Autodesk Fusion 360 part; units mm, degrees
(part 7 of 25)
  arc A2551 (12.8651, 8.7313) -> (12.8651, 8.6677) centre (12.8651, 8.6995) ccw
  line L798 (13.8532, 8.0645) -> (13.8532, 9.2075)
  arc A2552 (15.5982, 8.6789) -> (15.5498, 8.7201) centre (15.574, 8.6995) ccw
  arc A2553 (13.3731, 8.0328) -> (13.3731, 8.0963) centre (13.3731, 8.0646) ccw
  arc A2554 (76.9971, 14.0193) -> (77.0539, 14.0477) centre (77.0255, 14.0335) ccw
  arc A2555 (13.8532, 9.2393) -> (13.8532, 9.1757) centre (13.8532, 9.2075) ccw
  arc A2556 (14.5199, 8.382) -> (14.4564, 8.382) centre (14.4881, 8.382) ccw
  line L799 (76.3905, 14.0335) -> (76.3905, 15.1765)
  arc A2557 (15.0041, 8.9633) -> (15.0645, 8.9437) centre (15.0343, 8.9535) ccw
  line L800 (15.0343, 8.0645) -> (15.6693, 8.0645)
  arc A2558 (76.708, 14.5415) -> (76.708, 15.1765) centre (76.708, 14.859) ccw
  arc A2559 (13.2461, 8.6677) -> (13.2461, 8.7313) centre (13.2461, 8.6995) ccw
  arc A2560 (10.8248, 9.6965) -> (10.5391, 9.9822) centre (10.5391, 9.6965) ccw
  arc A2561 (10.8566, 9.6965) -> (10.7931, 9.6964) centre (10.8249, 9.6965) ccw
  arc A2562 (76.4223, 15.1765) -> (76.3588, 15.1765) centre (76.3906, 15.1765) ccw
  arc A2563 (10.1596, 9.738) -> (10.22, 9.7184) centre (10.1898, 9.7282) ccw
  arc A2564 (10.7538, 9.4536) -> (10.7054, 9.4948) centre (10.7296, 9.4742) ccw
  arc A2565 (9.0869, 9.9822) -> (9.0234, 9.9822) centre (9.0552, 9.9822) ccw
  arc A2566 (10.7296, 9.4742) -> (10.8248, 9.6965) centre (10.5179, 9.6964) ccw
  arc A2567 (10.5391, 9.9505) -> (10.5391, 10.014) centre (10.5391, 9.9823) ccw
  arc A2568 (77.9062, 28.2892) -> (77.9062, 28.2258) centre (77.9062, 28.2575) ccw
  arc A2569 (10.5391, 9.9822) -> (10.1898, 9.7282) centre (10.5391, 9.6151) ccw
  arc A2570 (10.7077, 9.4972) -> (10.7515, 9.4512) centre (10.7296, 9.4742) ccw
  line L801 (77.0255, 14.0335) -> (76.7715, 14.5415)
  arc A2571 (77.5252, 14.0653) -> (77.5252, 14.0017) centre (77.5252, 14.0335) ccw
  arc A2572 (10.5391, 10.014) -> (10.5391, 9.9505) centre (10.5391, 9.9823) ccw
  arc A2573 (76.708, 28.2258) -> (76.708, 28.2892) centre (76.708, 28.2575) ccw
  arc A2574 (9.0551, 9.379) -> (9.0551, 9.3155) centre (9.0551, 9.3473) ccw
  line L802 (77.5252, 27.1145) -> (77.8427, 27.1145)
  arc A2575 (77.5252, 28.2892) -> (77.5252, 28.2258) centre (77.5252, 28.2575) ccw
  arc A2576 (77.8427, 27.1145) -> (77.8427, 27.7495) centre (77.8427, 27.432) ccw
  arc A2577 (76.708, 27.6543) -> (76.708, 27.5908) centre (76.708, 27.6226) ccw
  arc A2578 (76.708, 27.5908) -> (76.708, 27.6543) centre (76.708, 27.6226) ccw
  arc A2579 (77.8625, 15.1517) -> (77.8229, 15.2013) centre (77.8427, 15.1765) ccw
  line L803 (76.708, 27.6225) -> (76.3905, 27.6225)
  arc A2580 (10.1898, 8.871) -> (10.1898, 8.8074) centre (10.1898, 8.8392) ccw
  arc A2581 (9.0551, 10.014) -> (9.0551, 9.9505) centre (9.0551, 9.9823) ccw
  arc A2582 (9.0234, 8.8392) -> (9.0869, 8.8392) centre (9.0552, 8.8392) ccw
  line L804 (77.9062, 27.7495) -> (77.6522, 27.7495)
  arc A2583 (77.9062, 28.2258) -> (77.9062, 28.2892) centre (77.9062, 28.2575) ccw
  arc A2584 (76.9971, 27.1003) -> (77.0539, 27.1287) centre (77.0255, 27.1145) ccw
  line L805 (9.3726, 9.3472) -> (9.0551, 9.3472)
  arc A2585 (77.811, 14.0335) -> (77.8745, 14.0335) centre (77.8428, 14.0335) ccw
  arc A2586 (9.3726, 9.379) -> (9.3726, 9.3155) centre (9.3726, 9.3473) ccw
  line L806 (76.3905, 27.1145) -> (76.3905, 28.2575)
  arc A2587 (9.3726, 9.3155) -> (9.3726, 9.379) centre (9.3726, 9.3473) ccw
  arc A2588 (76.7999, 27.6367) -> (76.7431, 27.6083) centre (76.7715, 27.6225) ccw
  arc A2589 (77.8427, 27.0828) -> (77.8427, 27.1462) centre (77.8427, 27.1145) ccw
  arc A2590 (77.8427, 27.1462) -> (77.8427, 27.0828) centre (77.8427, 27.1145) ccw
  arc A2591 (9.6617, 8.825) -> (9.7185, 8.8534) centre (9.6901, 8.8392) ccw
  arc A2592 (77.9062, 27.7178) -> (77.9062, 27.7813) centre (77.9062, 27.7496) ccw
  line L807 (10.7296, 9.4742) -> (10.1898, 8.8392)
  arc A2593 (76.3905, 28.2892) -> (76.3905, 28.2258) centre (76.3905, 28.2575) ccw
  arc A2594 (76.708, 28.2892) -> (76.708, 28.2258) centre (76.708, 28.2575) ccw
  line L808 (10.1898, 8.8392) -> (10.8248, 8.8392)
  line L809 (77.5252, 28.2575) -> (77.9062, 28.2575)
  line L810 (9.0551, 8.8392) -> (9.0551, 9.9822)
  line L811 (9.0551, 9.9822) -> (9.3726, 9.9822)
  arc A2595 (9.3726, 9.9505) -> (9.3726, 10.014) centre (9.3726, 9.9823) ccw
  line L812 (9.6901, 8.8392) -> (9.4361, 9.3472)
  arc A2596 (9.3726, 10.014) -> (9.3726, 9.9505) centre (9.3726, 9.9823) ccw
  line L813 (77.8427, 15.1765) -> (77.8427, 14.0335)
  arc A2597 (10.1656, 8.8598) -> (10.214, 8.8186) centre (10.1898, 8.8392) ccw
  arc A2598 (76.708, 15.2083) -> (76.708, 15.1448) centre (76.708, 15.1766) ccw
  arc A2599 (76.708, 14.5733) -> (76.708, 14.5098) centre (76.708, 14.5416) ccw
  arc A2600 (10.8248, 8.8074) -> (10.8248, 8.871) centre (10.8248, 8.8392) ccw
  arc A2601 (9.3726, 9.3472) -> (9.3726, 9.9822) centre (9.3726, 9.6647) ccw
  arc A2602 (76.3588, 27.1145) -> (76.4223, 27.1145) centre (76.3906, 27.1145) ccw
  arc A2603 (10.7931, 9.6965) -> (10.8566, 9.6965) centre (10.8249, 9.6965) ccw
  arc A2604 (77.9062, 27.7495) -> (77.9062, 28.2575) centre (77.9062, 28.0035) ccw
  arc A2605 (77.9062, 27.7813) -> (77.9062, 27.7178) centre (77.9062, 27.7496) ccw
  arc A2606 (9.4645, 9.3614) -> (9.4077, 9.333) centre (9.4361, 9.3472) ccw
  arc A2607 (77.6522, 27.7813) -> (77.6522, 27.7178) centre (77.6522, 27.7496) ccw
  arc A2608 (64.633, 27.136) -> (64.5729, 27.1565) centre (64.603, 27.1462) ccw
  arc A2609 (62.611, 23.0188) -> (62.611, 23.0822) centre (62.611, 23.0505) ccw
  arc A2610 (63.9362, 23.0188) -> (63.9362, 23.0822) centre (63.9362, 23.0505) ccw
  line L814 (64.1267, 27.2415) -> (64.6347, 27.8765)
  line L815 (63.2377, 28.1305) -> (63.2377, 26.9875)
  arc A2611 (63.3965, 22.5425) -> (63.46, 22.5425) centre (63.4283, 22.5425) ccw
  arc A2612 (77.5252, 27.1462) -> (77.5252, 27.0828) centre (77.5252, 27.1145) ccw
  arc A2613 (63.46, 22.5425) -> (63.3965, 22.5425) centre (63.4283, 22.5425) ccw
  line L816 (62.9285, 21.9075) -> (62.6745, 22.4155)
  arc A2614 (63.8092, 22.5742) -> (63.8092, 22.5108) centre (63.8092, 22.5425) ccw
  arc A2615 (76.4223, 28.2575) -> (76.3588, 28.2575) centre (76.3906, 28.2575) ccw
  arc A2616 (62.611, 22.4155) -> (62.611, 23.0505) centre (62.611, 22.733) ccw
  arc A2617 (63.4282, 22.225) -> (64.0632, 22.225) centre (63.7457, 22.225) ccw
  line L817 (61.7855, 26.9875) -> (61.7855, 28.1305)
  arc A2618 (64.5729, 27.9615) -> (64.633, 27.982) centre (64.603, 27.9718) ccw
  arc A2619 (62.611, 23.0822) -> (62.611, 23.0188) centre (62.611, 23.0505) ccw
  line L818 (63.4282, 22.225) -> (63.4282, 22.5425)
  arc A2620 (64.6315, 27.9857) -> (64.5744, 27.9578) centre (64.603, 27.9717) ccw
  arc A2621 (62.7029, 22.4297) -> (62.6461, 22.4013) centre (62.6745, 22.4155) ccw
  arc A2622 (64.095, 27.559) -> (64.0315, 27.559) centre (64.0632, 27.559) ccw
  arc A2623 (62.2935, 23.0822) -> (62.2935, 23.0188) centre (62.2935, 23.0505) ccw
  arc A2624 (62.9001, 21.8933) -> (62.9569, 21.9217) centre (62.9285, 21.9075) ccw
  line L819 (64.0632, 22.2885) -> (64.0632, 22.225)
  arc A2625 (62.2935, 22.4473) -> (62.2935, 22.3838) centre (62.2935, 22.4156) ccw
  arc A2626 (63.4282, 22.5742) -> (63.4282, 22.5108) centre (63.4282, 22.5425) ccw
  line L820 (63.4282, 22.5425) -> (63.8092, 22.5425)
  arc A2627 (62.2617, 21.9075) -> (62.3253, 21.9075) centre (62.2935, 21.9075) ccw
  arc A2628 (62.3253, 23.0505) -> (62.2617, 23.0505) centre (62.2935, 23.0505) ccw
  arc A2629 (64.0632, 27.559) -> (64.1585, 27.1463) centre (65.0049, 27.5591) ccw
  arc A2630 (64.0632, 22.2885) -> (63.8092, 22.5425) centre (63.8092, 22.2885) ccw
  arc A2631 (64.5744, 27.1602) -> (64.6315, 27.1323) centre (64.603, 27.1463) ccw
  arc A2632 (64.187, 27.9578) -> (64.1299, 27.9857) centre (64.1585, 27.9717) ccw
  arc A2633 (64.603, 27.1463) -> (64.6982, 27.559) centre (63.7565, 27.5589) ccw
  arc A2634 (64.3807, 26.9875) -> (64.603, 27.1463) centre (64.3807, 27.2225) ccw
  arc A2635 (63.9362, 23.0505) -> (63.4282, 22.5425) centre (63.9362, 22.5425) ccw
  arc A2636 (64.1299, 27.1323) -> (64.187, 27.1602) centre (64.1585, 27.1462) ccw
  arc A2637 (63.3965, 22.225) -> (63.46, 22.225) centre (63.4283, 22.225) ccw
  line L821 (62.4205, 26.9875) -> (62.1665, 27.4955)
  line L822 (62.2935, 21.9075) -> (62.2935, 23.0505)
  arc A2638 (63.8092, 22.5108) -> (63.8092, 22.5742) centre (63.8092, 22.5425) ccw
  line L823 (76.3905, 28.2575) -> (76.708, 28.2575)
  arc A2639 (63.46, 22.225) -> (63.3965, 22.225) centre (63.4283, 22.225) ccw
  arc A2640 (64.095, 22.225) -> (64.0315, 22.225) centre (64.0632, 22.225) ccw
  line L824 (62.611, 22.4155) -> (62.2935, 22.4155)
  arc A2641 (62.611, 22.3838) -> (62.611, 22.4473) centre (62.611, 22.4156) ccw
  arc A2642 (77.8427, 27.7813) -> (77.8427, 27.7178) centre (77.8427, 27.7496) ccw
  arc A2643 (64.1284, 27.982) -> (64.1885, 27.9615) centre (64.1585, 27.9717) ccw
  arc A2644 (64.095, 22.2885) -> (64.0315, 22.2885) centre (64.0632, 22.2885) ccw
  arc A2645 (62.9004, 27.9013) -> (62.94, 27.8517) centre (62.9202, 27.8765) ccw
  arc A2646 (61.7855, 27.5272) -> (61.7855, 27.4638) centre (61.7855, 27.4955) ccw
  arc A2647 (63.5552, 26.9558) -> (63.5552, 27.0192) centre (63.5552, 26.9875) ccw
  arc A2648 (76.708, 27.6225) -> (76.708, 28.2575) centre (76.708, 27.94) ccw
  arc A2649 (62.611, 22.4473) -> (62.611, 22.3838) centre (62.611, 22.4156) ccw
  line L825 (77.0255, 27.1145) -> (76.7715, 27.6225)
  arc A2650 (64.0315, 22.2885) -> (64.095, 22.2885) centre (64.0632, 22.2885) ccw
  arc A2651 (64.3807, 26.9558) -> (64.3807, 27.0192) centre (64.3807, 26.9875) ccw
  line L826 (61.7855, 28.1305) -> (62.103, 28.1305)
  arc A2652 (62.103, 28.0988) -> (62.103, 28.1623) centre (62.103, 28.1305) ccw
  arc A2653 (61.7538, 26.9875) -> (61.8173, 26.9875) centre (61.7856, 26.9875) ccw
  arc A2654 (76.3905, 27.6543) -> (76.3905, 27.5908) centre (76.3905, 27.6226) ccw
  arc A2655 (64.0315, 22.225) -> (64.095, 22.225) centre (64.0632, 22.225) ccw
  line L827 (62.2935, 23.0505) -> (62.611, 23.0505)
  arc A2656 (62.1949, 27.5097) -> (62.1381, 27.4813) centre (62.1665, 27.4955) ccw
  arc A2657 (44.577, 36.0998) -> (44.577, 36.1633) centre (44.577, 36.1316) ccw
  arc A2658 (64.0315, 27.559) -> (64.095, 27.559) centre (64.0632, 27.559) ccw
  line L828 (44.8945, 35.6235) -> (44.6405, 36.1315)
  arc A2659 (44.577, 36.7347) -> (44.577, 36.7983) centre (44.577, 36.7665) ccw
  arc A2660 (45.7315, 36.7417) -> (45.6919, 36.7913) centre (45.7117, 36.7665) ccw
  arc A2661 (44.2595, 36.7983) -> (44.2595, 36.7347) centre (44.2595, 36.7665) ccw
  line L829 (62.9202, 27.8765) -> (63.2377, 28.1305)
  line L830 (62.9202, 26.9875) -> (63.5552, 26.9875)
  arc A2662 (61.7855, 28.1623) -> (61.7855, 28.0988) centre (61.7855, 28.1305) ccw
  line L831 (44.2595, 35.6235) -> (44.2595, 36.7665)
  line L832 (44.577, 36.1315) -> (44.2595, 36.1315)
  line L833 (46.5372, 35.6235) -> (46.8547, 35.6235)
  arc A2663 (44.2595, 36.1633) -> (44.2595, 36.0998) centre (44.2595, 36.1316) ccw
  arc A2664 (64.1585, 27.1463) -> (64.3807, 26.9875) centre (64.3807, 27.2224) ccw
  arc A2665 (64.6595, 27.8567) -> (64.6099, 27.8963) centre (64.6347, 27.8765) ccw
  arc A2666 (64.3807, 28.1305) -> (64.1585, 27.9718) centre (64.3807, 27.8956) ccw
  arc A2667 (44.6322, 30.3848) -> (44.6322, 30.4483) centre (44.6322, 30.4166) ccw
  arc A2668 (45.3744, 36.5373) -> (45.414, 36.4877) centre (45.3942, 36.5125) ccw
  arc A2669 (46.5372, 35.6553) -> (46.5372, 35.5917) centre (46.5372, 35.6235) ccw
  arc A2670 (44.6689, 36.1457) -> (44.6121, 36.1173) centre (44.6405, 36.1315) ccw
  arc A2671 (45.68, 35.6235) -> (45.7435, 35.6235) centre (45.7118, 35.6235) ccw
  arc A2672 (44.2278, 35.6235) -> (44.2913, 35.6235) centre (44.2596, 35.6235) ccw
  arc A2673 (62.103, 27.5272) -> (62.103, 27.4638) centre (62.103, 27.4955) ccw
  arc A2674 (64.3807, 28.0988) -> (64.3807, 28.1623) centre (64.3807, 28.1305) ccw
  line L834 (44.3147, 31.5595) -> (44.3147, 30.4165)
  arc A2675 (64.3807, 28.1623) -> (64.3807, 28.0988) centre (64.3807, 28.1305) ccw
  arc A2676 (64.3807, 27.0192) -> (64.3807, 26.9558) centre (64.3807, 26.9875) ccw
  arc A2677 (62.3921, 26.9733) -> (62.4489, 27.0017) centre (62.4205, 26.9875) ccw
  arc A2678 (64.73, 27.559) -> (64.6665, 27.559) centre (64.6983, 27.559) ccw
  arc A2679 (46.0292, 35.5917) -> (46.0292, 35.6553) centre (46.0292, 35.6235) ccw
  arc A2680 (46.8547, 35.6235) -> (46.8547, 36.2585) centre (46.8547, 35.941) ccw
  arc A2681 (62.9202, 27.0192) -> (62.9202, 26.9558) centre (62.9202, 26.9875) ccw
  arc A2682 (63.206, 26.9875) -> (63.2695, 26.9875) centre (63.2378, 26.9875) ccw
  arc A2683 (64.603, 27.9718) -> (64.3807, 28.1305) centre (64.3808, 27.8956) ccw
  arc A2684 (61.8173, 28.1305) -> (61.7538, 28.1305) centre (61.7856, 28.1305) ccw
  arc A2685 (44.8661, 35.6093) -> (44.9229, 35.6377) centre (44.8945, 35.6235) ccw
  arc A2686 (63.2575, 28.1057) -> (63.2179, 28.1553) centre (63.2377, 28.1305) ccw
  line L835 (45.3942, 36.5125) -> (45.7117, 36.7665)
  arc A2687 (63.2695, 28.1305) -> (63.206, 28.1305) centre (63.2378, 28.1305) ccw
  arc A2688 (62.103, 28.1623) -> (62.103, 28.0988) centre (62.103, 28.1305) ccw
  line L836 (45.7117, 36.7665) -> (45.7117, 35.6235)
  arc A2689 (64.1585, 27.9718) -> (64.0632, 27.559) centre (65.0052, 27.5589) ccw
  arc A2690 (45.3942, 35.6553) -> (45.3942, 35.5917) centre (45.3942, 35.6235) ccw
  arc A2691 (45.7435, 36.7665) -> (45.68, 36.7665) centre (45.7118, 36.7665) ccw
  arc A2692 (64.1019, 27.2613) -> (64.1515, 27.2217) centre (64.1267, 27.2415) ccw
  arc A2693 (62.103, 27.4638) -> (62.103, 27.5272) centre (62.103, 27.4955) ccw
  arc A2694 (64.1885, 27.1565) -> (64.1284, 27.136) centre (64.1585, 27.1462) ccw
  arc A2695 (43.9972, 30.4483) -> (43.9972, 30.3848) centre (43.9972, 30.4166) ccw
  arc A2696 (44.577, 36.1633) -> (44.577, 36.0998) centre (44.577, 36.1316) ccw
  line L837 (44.2595, 36.7665) -> (44.577, 36.7665)
  arc A2697 (44.577, 36.7983) -> (44.577, 36.7347) centre (44.577, 36.7665) ccw
  arc A2698 (44.2913, 36.7665) -> (44.2278, 36.7665) centre (44.2596, 36.7665) ccw
  arc A2699 (62.103, 27.4955) -> (62.103, 28.1305) centre (62.103, 27.813) ccw
  line L838 (45.3942, 35.6235) -> (46.0292, 35.6235)
  arc A2700 (46.8547, 35.5917) -> (46.8547, 35.6553) centre (46.8547, 35.6235) ccw
  arc A2701 (64.6665, 27.559) -> (64.73, 27.559) centre (64.6983, 27.559) ccw
  line L839 (62.103, 27.4955) -> (61.7855, 27.4955)
  arc A2702 (44.577, 36.1315) -> (44.577, 36.7665) centre (44.577, 36.449) ccw
  arc A2703 (64.6982, 27.559) -> (64.603, 27.9718) centre (63.7563, 27.5592) ccw
  arc A2704 (46.9182, 36.7983) -> (46.9182, 36.7347) centre (46.9182, 36.7665) ccw
  arc A2705 (44.323, 44.6088) -> (44.323, 44.6723) centre (44.323, 44.6406) ccw
  arc A2706 (44.0055, 44.6723) -> (44.0055, 44.6088) centre (44.0055, 44.6406) ccw
  arc A2707 (45.1402, 43.5293) -> (45.1402, 43.4657) centre (45.1402, 43.4975) ccw
  arc A2708 (46.9182, 43.7197) -> (46.9182, 43.7833) centre (46.9182, 43.7515) ccw
  arc A2709 (46.696, 43.4975) -> (46.7595, 43.4975) centre (46.7278, 43.4975) ccw
  arc A2710 (46.9182, 36.2585) -> (46.9182, 36.7665) centre (46.9182, 36.5125) ccw
  line L840 (31.1702, 44.3865) -> (31.4877, 44.6405)
  arc A2711 (30.4449, 44.0197) -> (30.3881, 43.9913) centre (30.4165, 44.0055) ccw
  arc A2712 (30.6421, 43.4833) -> (30.6989, 43.5117) centre (30.6705, 43.4975) ccw
  arc A2713 (31.5075, 44.6157) -> (31.4679, 44.6653) centre (31.4877, 44.6405) ccw
  arc A2714 (45.4775, 44.6157) -> (45.4379, 44.6653) centre (45.4577, 44.6405) ccw
  line L841 (45.4577, 44.6405) -> (45.4577, 43.4975)
  line L842 (44.323, 44.0055) -> (44.0055, 44.0055)
  arc A2715 (44.0055, 44.0373) -> (44.0055, 43.9738) centre (44.0055, 44.0055) ccw
  arc A2716 (44.4149, 44.0197) -> (44.3581, 43.9913) centre (44.3865, 44.0055) ccw
  arc A2717 (43.9738, 43.4975) -> (44.0373, 43.4975) centre (44.0055, 43.4975) ccw
  arc A2718 (44.323, 44.0373) -> (44.323, 43.9738) centre (44.323, 44.0055) ccw
  arc A2719 (46.9182, 36.7347) -> (46.9182, 36.7983) centre (46.9182, 36.7665) ccw
  arc A2720 (46.8547, 35.6553) -> (46.8547, 35.5917) centre (46.8547, 35.6235) ccw
  arc A2721 (46.9182, 36.2268) -> (46.9182, 36.2903) centre (46.9182, 36.2585) ccw
  arc A2722 (44.6121, 43.4833) -> (44.6689, 43.5117) centre (44.6405, 43.4975) ccw
  arc A2723 (44.323, 43.9738) -> (44.323, 44.0373) centre (44.323, 44.0055) ccw
  arc A2724 (45.4895, 44.6405) -> (45.426, 44.6405) centre (45.4577, 44.6405) ccw
  arc A2725 (46.2832, 43.7833) -> (46.2832, 43.7197) centre (46.2832, 43.7515) ccw
  line L843 (44.6405, 43.4975) -> (44.3865, 44.0055)
  arc A2726 (46.9182, 36.2903) -> (46.9182, 36.2268) centre (46.9182, 36.2585) ccw
  line L844 (46.5372, 44.6405) -> (46.2832, 43.7515)
  arc A2727 (30.0355, 44.0373) -> (30.0355, 43.9738) centre (30.0355, 44.0055) ccw
  arc A2728 (30.0355, 44.6723) -> (30.0355, 44.6088) centre (30.0355, 44.6406) ccw
  line L845 (44.0055, 44.6405) -> (44.323, 44.6405)
  line L846 (45.1402, 44.3865) -> (45.4577, 44.6405)
  arc A2729 (46.8547, 36.2903) -> (46.8547, 36.2268) centre (46.8547, 36.2585) ccw
  arc A2730 (46.5372, 36.7983) -> (46.5372, 36.7347) centre (46.5372, 36.7665) ccw
  arc A2731 (46.5677, 44.6318) -> (46.5067, 44.6492) centre (46.5372, 44.6405) ccw
  line L847 (46.2832, 43.7515) -> (46.9182, 43.7515)
  line L848 (46.9182, 36.2585) -> (46.6642, 36.2585)
  arc A2732 (31.1504, 44.4113) -> (31.19, 44.3617) centre (31.1702, 44.3865) ccw
  arc A2733 (46.2527, 43.7602) -> (46.3137, 43.7428) centre (46.2832, 43.7515) ccw
  line L849 (31.4877, 44.6405) -> (31.4877, 43.4975)
  arc A2734 (45.7752, 43.4657) -> (45.7752, 43.5293) centre (45.7752, 43.4975) ccw
  arc A2735 (44.323, 44.6723) -> (44.323, 44.6088) centre (44.323, 44.6406) ccw
  arc A2736 (31.5195, 44.6405) -> (31.456, 44.6405) centre (31.4878, 44.6405) ccw
  line L850 (46.7277, 44.0055) -> (46.7277, 43.4975)
  line L851 (31.1702, 43.4975) -> (31.8052, 43.4975)
  line L852 (46.5372, 36.7665) -> (46.9182, 36.7665)
  arc A2737 (44.0373, 44.6405) -> (43.9738, 44.6405) centre (44.0055, 44.6405) ccw
  arc A2738 (46.7595, 44.0055) -> (46.696, 44.0055) centre (46.7278, 44.0055) ccw
  arc A2739 (45.1204, 44.4113) -> (45.16, 44.3617) centre (45.1402, 44.3865) ccw
  arc A2740 (30.353, 44.6723) -> (30.353, 44.6088) centre (30.353, 44.6406) ccw
  line L853 (30.6705, 43.4975) -> (30.4165, 44.0055)
  arc A2741 (45.426, 43.4975) -> (45.4895, 43.4975) centre (45.4577, 43.4975) ccw
  arc A2742 (30.0673, 44.6405) -> (30.0038, 44.6405) centre (30.0356, 44.6405) ccw
  line L854 (45.1402, 43.4975) -> (45.7752, 43.4975)
  arc A2743 (46.6642, 36.2903) -> (46.6642, 36.2268) centre (46.6642, 36.2585) ccw
  line L855 (44.0055, 43.4975) -> (44.0055, 44.6405)
  arc A2744 (30.353, 43.9738) -> (30.353, 44.0373) centre (30.353, 44.0055) ccw
  arc A2745 (30.0038, 43.4975) -> (30.0673, 43.4975) centre (30.0356, 43.4975) ccw
  arc A2746 (31.456, 43.4975) -> (31.5195, 43.4975) centre (31.4878, 43.4975) ccw
  line L856 (30.353, 44.0055) -> (30.0355, 44.0055)
  arc A2747 (44.323, 44.0055) -> (44.323, 44.6405) centre (44.323, 44.323) ccw
  line L857 (30.0355, 44.6405) -> (30.353, 44.6405)
  arc A2748 (8.763, 17.1768) -> (8.763, 17.2402) centre (8.763, 17.2085) ccw
  arc A2749 (8.8549, 17.2227) -> (8.7981, 17.1943) centre (8.8265, 17.2085) ccw
  arc A2750 (11.39, 17.018) -> (11.3265, 17.018) centre (11.3582, 17.018) ccw
  arc A2751 (9.5604, 17.6143) -> (9.6, 17.5647) centre (9.5802, 17.5895) ccw
  arc A2752 (10.6915, 17.3355) -> (10.755, 17.3355) centre (10.7233, 17.3355) ccw
  line L858 (32.3132, 44.1325) -> (32.3132, 44.6405)
  arc A2753 (32.6942, 43.4975) -> (32.9482, 43.7515) centre (32.6942, 43.7515) ccw
  arc A2754 (32.9165, 43.7515) -> (32.98, 43.7515) centre (32.9483, 43.7515) ccw
  arc A2755 (8.763, 17.2085) -> (8.763, 17.8435) centre (8.763, 17.526) ccw
  arc A2756 (32.98, 43.7515) -> (32.9165, 43.7515) centre (32.9483, 43.7515) ccw
  line L859 (32.3132, 43.4975) -> (32.6942, 43.4975)
  arc A2757 (82.3874, 4.699) -> (82.6414, 4.953) centre (82.3874, 4.953) ccw
  arc A2758 (30.353, 44.0373) -> (30.353, 43.9738) centre (30.353, 44.0055) ccw
  arc A2759 (32.6942, 43.5293) -> (32.6942, 43.4657) centre (32.6942, 43.4975) ccw
  arc A2760 (32.345, 44.6405) -> (32.2815, 44.6405) centre (32.3133, 44.6405) ccw
  line L860 (9.0805, 16.7005) -> (8.8265, 17.2085)
  line L861 (11.3582, 17.0815) -> (11.3582, 17.018)
  arc A2761 (31.1702, 43.5293) -> (31.1702, 43.4657) centre (31.1702, 43.4975) ccw
  arc A2762 (31.8052, 43.4657) -> (31.8052, 43.5293) centre (31.8052, 43.4975) ccw
  arc A2763 (9.9295, 17.8435) -> (9.866, 17.8435) centre (9.8978, 17.8435) ccw
  arc A2764 (11.39, 17.0815) -> (11.3265, 17.0815) centre (11.3582, 17.0815) ccw
  arc A2765 (9.866, 16.7005) -> (9.9295, 16.7005) centre (9.8978, 16.7005) ccw
  arc A2766 (30.353, 44.0055) -> (30.353, 44.6405) centre (30.353, 44.323) ccw
  arc A2767 (32.6942, 43.4657) -> (32.6942, 43.5293) centre (32.6942, 43.4975) ccw
  line L862 (9.5802, 16.7005) -> (10.2152, 16.7005)
  line L863 (10.7232, 17.018) -> (10.7232, 17.3355)
  line L864 (9.5802, 17.5895) -> (9.8977, 17.8435)
  arc A2768 (8.4773, 17.8435) -> (8.4138, 17.8435) centre (8.4456, 17.8435) ccw
  arc A2769 (9.5802, 16.7323) -> (9.5802, 16.6688) centre (9.5802, 16.7005) ccw
  line L865 (10.7232, 17.3355) -> (11.1042, 17.3355)
  line L866 (30.0355, 43.4975) -> (30.0355, 44.6405)
  line L867 (32.3132, 44.6405) -> (32.9482, 44.6405)
  arc A2770 (11.3265, 17.0815) -> (11.39, 17.0815) centre (11.3582, 17.0815) ccw
  arc A2771 (32.2815, 44.1325) -> (32.345, 44.1325) centre (32.3133, 44.1325) ccw
  arc A2772 (8.4138, 16.7005) -> (8.4773, 16.7005) centre (8.4456, 16.7005) ccw
  arc A2773 (30.353, 44.6088) -> (30.353, 44.6723) centre (30.353, 44.6406) ccw
  arc A2774 (32.3132, 44.6723) -> (32.3132, 44.6088) centre (32.3132, 44.6406) ccw
  arc A2775 (32.98, 43.8785) -> (32.9165, 43.8785) centre (32.9483, 43.8785) ccw
  arc A2776 (8.4455, 17.8753) -> (8.4455, 17.8118) centre (8.4455, 17.8436) ccw
  arc A2777 (32.9165, 43.8785) -> (32.98, 43.8785) centre (32.9483, 43.8785) ccw
  arc A2778 (32.6942, 44.1643) -> (32.6942, 44.1007) centre (32.6942, 44.1325) ccw
  arc A2779 (8.4455, 17.2402) -> (8.4455, 17.1768) centre (8.4455, 17.2085) ccw
  arc A2780 (9.9175, 17.8187) -> (9.8779, 17.8683) centre (9.8977, 17.8435) ccw
  arc A2781 (10.7232, 17.3672) -> (10.7232, 17.3038) centre (10.7232, 17.3355) ccw
  arc A2782 (32.3132, 43.5293) -> (32.3132, 43.4657) centre (32.3132, 43.4975) ccw
  arc A2783 (10.755, 17.018) -> (10.6915, 17.018) centre (10.7233, 17.018) ccw
  arc A2784 (10.755, 17.3355) -> (10.6915, 17.3355) centre (10.7233, 17.3355) ccw
  line L868 (8.4455, 16.7005) -> (8.4455, 17.8435)
  arc A2785 (32.9482, 43.8785) -> (32.6942, 44.1325) centre (32.6942, 43.8785) ccw
  line L869 (8.763, 17.2085) -> (8.4455, 17.2085)
  arc A2786 (32.9482, 44.6088) -> (32.9482, 44.6723) centre (32.9482, 44.6406) ccw
  line L870 (32.6942, 44.1325) -> (32.3132, 44.1325)
  line L871 (32.9482, 43.7515) -> (32.9482, 43.8785)
  line L872 (8.4455, 17.8435) -> (8.763, 17.8435)
  arc A2787 (8.763, 17.8753) -> (8.763, 17.8118) centre (8.763, 17.8436) ccw
  arc A2788 (10.2152, 16.6688) -> (10.2152, 16.7323) centre (10.2152, 16.7005) ccw
  arc A2789 (32.3132, 44.1643) -> (32.3132, 44.1007) centre (32.3132, 44.1325) ccw
  arc A2790 (11.3265, 17.018) -> (11.39, 17.018) centre (11.3582, 17.018) ccw
  arc A2791 (32.6942, 44.1007) -> (32.6942, 44.1643) centre (32.6942, 44.1325) ccw
  arc A2792 (10.7232, 17.018) -> (11.3582, 17.018) centre (11.0407, 17.018) ccw
  arc A2793 (8.763, 17.2402) -> (8.763, 17.1768) centre (8.763, 17.2085) ccw
  arc A2794 (8.763, 17.8118) -> (8.763, 17.8753) centre (8.763, 17.8436) ccw
  arc A2795 (11.2312, 17.8118) -> (11.2312, 17.8753) centre (11.2312, 17.8436) ccw
  line L873 (9.8977, 17.8435) -> (9.8977, 16.7005)
  arc A2796 (9.0521, 16.6863) -> (9.1089, 16.7147) centre (9.0805, 16.7005) ccw
  arc A2797 (82.4992, 5.1474) -> (82.5296, 5.2031) centre (82.5144, 5.1753) ccw
  arc A2798 (82.3595, 18.6055) -> (82.6135, 18.8595) centre (82.3595, 18.8595) ccw
  arc A2799 (82.4713, 19.0539) -> (82.5017, 19.1096) centre (82.4865, 19.0817) ccw
  arc A2800 (83.4326, 19.7168) -> (83.4327, 19.7802) centre (83.4326, 19.7485) ccw
  arc A2801 (83.0915, 5.6128) -> (83.1312, 5.5632) centre (83.1114, 5.588) ccw
  arc A2802 (82.5309, 19.6279) -> (82.5691, 19.6786) centre (82.55, 19.6532) ccw
  arc A2803 (82.1804, 5.3936) -> (82.15, 5.3379) centre (82.1652, 5.3657) ccw
  arc A2804 (82.5026, 19.1091) -> (82.4704, 19.0544) centre (82.4865, 19.0817) ccw
  line L874 (83.1113, 5.588) -> (83.4288, 5.842)
  arc A2805 (82.0699, 5.588) -> (82.0064, 5.588) centre (82.0382, 5.588) ccw
  line L875 (82.5144, 5.1753) -> (82.1652, 5.3658)
  arc A2806 (82.0064, 4.8578) -> (82.3874, 4.699) centre (82.3875, 5.2356) ccw
  arc A2807 (83.7463, 4.6673) -> (83.7463, 4.7307) centre (83.7463, 4.699) ccw
  arc A2808 (82.3595, 18.6372) -> (82.3595, 18.5738) centre (82.3595, 18.6055) ccw
  arc A2809 (83.4487, 5.8172) -> (83.409, 5.8668) centre (83.4289, 5.842) ccw
  arc A2810 (82.3874, 4.7307) -> (82.3874, 4.6673) centre (82.3874, 4.699) ccw
  arc A2811 (83.0592, 18.6261) -> (83.1076, 18.5849) centre (83.0834, 18.6055) ccw
  arc A2812 (82.6097, 4.953) -> (82.6732, 4.953) centre (82.6414, 4.953) ccw
  arc A2813 (82.2643, 19.7485) -> (82.0102, 19.4945) centre (82.2643, 19.4944) ccw
  arc A2814 (83.4327, 19.7802) -> (83.4327, 19.7168) centre (83.4327, 19.7485) ccw
  arc A2815 (83.7501, 19.4628) -> (83.6867, 19.4627) centre (83.7184, 19.4628) ccw
  arc A2816 (83.3971, 4.699) -> (83.4606, 4.699) centre (83.4288, 4.699) ccw
  arc A2817 (82.5779, 5.7468) -> (82.2922, 5.842) centre (82.2923, 5.3659) ccw
  arc A2818 (82.6453, 18.8595) -> (82.5817, 18.8595) centre (82.6135, 18.8595) ccw
  arc A2819 (82.55, 19.6532) -> (82.2643, 19.7485) centre (82.2642, 19.2724) ccw
  arc A2820 (82.2643, 19.7168) -> (82.2643, 19.7802) centre (82.2643, 19.7485) ccw
  line L876 (83.6232, 19.2405) -> (83.0834, 18.6055)
  arc A2821 (83.6473, 19.2199) -> (83.599, 19.2611) centre (83.6232, 19.2405) ccw
  arc A2822 (83.0834, 18.6372) -> (83.0834, 18.5738) centre (83.0834, 18.6055) ccw
  arc A2823 (82.1211, 19.2449) -> (82.1534, 19.2996) centre (82.1372, 19.2723) ccw
  arc A2824 (82.3595, 18.5738) -> (82.3595, 18.6372) centre (82.3595, 18.6055) ccw
  arc A2825 (83.0532, 19.5043) -> (83.1136, 19.4847) centre (83.0834, 19.4945) ccw
  arc A2826 (82.1491, 5.3384) -> (82.1813, 5.3931) centre (82.1652, 5.3658) ccw
  line L877 (83.0834, 18.6055) -> (83.7184, 18.6055)
  arc A2827 (82.029, 4.8801) -> (81.9839, 4.8354) centre (82.0065, 4.8577) ccw
  arc A2828 (82.2922, 5.8738) -> (82.2922, 5.8103) centre (82.2922, 5.842) ccw
  arc A2829 (83.4606, 5.842) -> (83.3971, 5.842) centre (83.4288, 5.842) ccw
  arc A2830 (10.6915, 17.018) -> (10.755, 17.018) centre (10.7233, 17.018) ccw
  arc A2831 (82.6732, 4.953) -> (82.6097, 4.953) centre (82.6414, 4.953) ccw
  arc A2832 (82.0064, 5.588) -> (82.0699, 5.588) centre (82.0382, 5.588) ccw
  arc A2833 (83.6013, 19.2635) -> (83.645, 19.2175) centre (83.6231, 19.2405) ccw
  arc A2834 (82.2642, 19.7802) -> (82.2643, 19.7168) centre (82.2643, 19.7485) ccw
  arc A2835 (83.7184, 18.5738) -> (83.7184, 18.6372) centre (83.7184, 18.6055) ccw
  line L878 (83.1113, 4.699) -> (83.7463, 4.699)
  arc A2836 (82.0382, 5.588) -> (82.1652, 5.3658) centre (82.2961, 5.588) ccw
  arc A2837 (82.001, 18.7866) -> (81.956, 18.7419) centre (81.9785, 18.7643) ccw
  arc A2838 (83.4327, 19.7485) -> (83.0834, 19.4945) centre (83.4327, 19.3814) ccw
  arc A2839 (81.9785, 19.4945) -> (82.042, 19.4945) centre (82.0103, 19.4945) ccw
  arc A2840 (82.5306, 5.2026) -> (82.4983, 5.1479) centre (82.5145, 5.1753) ccw
  arc A2841 (82.2922, 5.842) -> (82.0382, 5.588) centre (82.2922, 5.588) ccw
  line L879 (83.4288, 5.842) -> (83.4288, 4.699)
  arc A2842 (82.5589, 5.7214) -> (82.597, 5.7721) centre (82.5779, 5.7468) ccw
  arc A2843 (11.1042, 17.3672) -> (11.1042, 17.3038) centre (11.1042, 17.3355) ccw
  arc A2844 (82.3874, 4.6673) -> (82.3874, 4.7307) centre (82.3874, 4.699) ccw
  arc A2845 (81.9785, 18.7643) -> (82.3595, 18.6055) centre (82.3596, 19.1421) ccw
  arc A2846 (11.1042, 17.3038) -> (11.1042, 17.3672) centre (11.1042, 17.3355) ccw
  arc A2847 (83.6867, 19.4627) -> (83.7502, 19.4627) centre (83.7185, 19.4627) ccw
  arc A2848 (11.2312, 17.8435) -> (10.7232, 17.3355) centre (11.2312, 17.3355) ccw
  arc A2849 (11.3582, 17.0815) -> (11.1042, 17.3355) centre (11.1042, 17.0815) ccw
  arc A2850 (82.2922, 5.8103) -> (82.2922, 5.8738) centre (82.2922, 5.842) ccw
  arc A2851 (82.6414, 4.953) -> (82.5144, 5.1753) centre (82.3834, 4.953) ccw
  arc A2852 (83.1113, 4.7307) -> (83.1113, 4.6673) centre (83.1113, 4.699) ccw
  line L880 (82.4865, 19.0817) -> (82.1373, 19.2722)
  arc A2853 (15.326, 27.5496) -> (15.281, 27.5049) centre (15.3035, 27.5273) ccw
  arc A2854 (15.875, 28.4163) -> (15.5893, 28.5115) centre (15.5894, 28.0354) ccw
  line L881 (16.7005, 28.5115) -> (17.0815, 28.5115)
  arc A2855 (15.4461, 28.0079) -> (15.4784, 28.0626) centre (15.4623, 28.0352) ccw
  arc A2856 (16.4782, 27.6225) -> (16.4148, 27.6225) centre (16.4465, 27.6225) ccw
  arc A2857 (17.6078, 28.2823) -> (17.6474, 28.2327) centre (17.6276, 28.2575) ccw
  line L882 (20.3073, 36.1315) -> (20.6248, 36.3855)
  arc A2858 (16.891, 28.0353) -> (16.891, 27.9718) centre (16.891, 28.0036) ccw
  line L883 (17.6276, 27.3685) -> (18.2626, 27.3685)
  arc A2859 (17.0815, 27.3368) -> (17.0815, 27.4002) centre (17.0815, 27.3685) ccw
  arc A2860 (15.9068, 27.6225) -> (15.9703, 27.6225) centre (15.9386, 27.6225) ccw
  arc A2861 (16.7005, 28.5115) -> (16.4465, 28.2575) centre (16.7005, 28.2575) ccw
  arc A2862 (15.4775, 28.0631) -> (15.447, 28.0074) centre (15.4622, 28.0353) ccw
  arc A2863 (17.0815, 28.4798) -> (17.0815, 28.5433) centre (17.0815, 28.5115) ccw
  arc A2864 (82.042, 19.4945) -> (81.9785, 19.4945) centre (82.0103, 19.4945) ccw
  arc A2865 (82.6135, 18.8595) -> (82.4865, 19.0817) centre (82.3556, 18.8595) ccw
  arc A2866 (82.1525, 19.3001) -> (82.122, 19.2444) centre (82.1372, 19.2723) ccw
  arc A2867 (16.4782, 28.2575) -> (16.4148, 28.2575) centre (16.4465, 28.2575) ccw
  arc A2868 (15.5892, 28.5433) -> (15.5893, 28.4798) centre (15.5893, 28.5115) ccw
  arc A2869 (17.0815, 27.9718) -> (17.0815, 28.0353) centre (17.0815, 28.0036) ccw
  arc A2870 (18.2626, 27.3368) -> (18.2626, 27.4002) centre (18.2626, 27.3685) ccw
  line L884 (20.6248, 36.3855) -> (20.6248, 35.2425)
  arc A2871 (15.3035, 27.5273) -> (15.6845, 27.3685) centre (15.6846, 27.9051) ccw
  arc A2872 (16.7005, 27.4002) -> (16.7005, 27.3368) centre (16.7005, 27.3685) ccw
  arc A2873 (15.3035, 28.2575) -> (15.367, 28.2575) centre (15.3353, 28.2575) ccw
  arc A2874 (82.0102, 19.4945) -> (82.1373, 19.2722) centre (82.2682, 19.4945) ccw
  line L885 (16.891, 28.0035) -> (17.0815, 28.0035)
  arc A2875 (15.5893, 28.4798) -> (15.5893, 28.5433) centre (15.5893, 28.5115) ccw
  arc A2876 (82.5817, 18.8595) -> (82.6453, 18.8595) centre (82.6135, 18.8595) ccw
  arc A2877 (15.6845, 27.3368) -> (15.6845, 27.4002) centre (15.6845, 27.3685) ccw
  arc A2878 (83.6232, 19.2405) -> (83.7184, 19.4627) centre (83.4116, 19.4626) ccw
  line L886 (19.558, 35.2425) -> (19.558, 36.3855)
  line L887 (16.4465, 27.6225) -> (16.4465, 28.2575)
  line L888 (17.0815, 28.0035) -> (17.0815, 27.3685)
  arc A2879 (19.5263, 35.2425) -> (19.5897, 35.2425) centre (19.558, 35.2425) ccw
  arc A2880 (20.6446, 36.3607) -> (20.605, 36.4103) centre (20.6248, 36.3855) ccw
  arc A2881 (20.2875, 36.1563) -> (20.3271, 36.1067) centre (20.3073, 36.1315) ccw
  arc A2882 (16.4465, 27.6225) -> (16.7005, 27.3685) centre (16.7005, 27.6225) ccw
  arc A2883 (15.9703, 27.6225) -> (15.9068, 27.6225) centre (15.9386, 27.6225) ccw
  arc A2884 (15.8559, 28.3909) -> (15.8941, 28.4416) centre (15.875, 28.4163) ccw
  arc A2885 (83.7184, 19.4627) -> (83.4327, 19.7485) centre (83.4326, 19.4627) ccw
  arc A2886 (17.9134, 27.3685) -> (17.9768, 27.3685) centre (17.9451, 27.3685) ccw
  arc A2887 (16.7005, 27.3368) -> (16.7005, 27.4002) centre (16.7005, 27.3685) ccw
  arc A2888 (15.5893, 28.5115) -> (15.3353, 28.2575) centre (15.5893, 28.2575) ccw
  arc A2889 (17.9649, 28.4867) -> (17.9253, 28.5363) centre (17.9451, 28.5115) ccw
  arc A2890 (20.6565, 36.3855) -> (20.5931, 36.3855) centre (20.6248, 36.3855) ccw
  line L889 (17.9451, 28.5115) -> (17.9451, 27.3685)
  line L890 (19.2405, 36.3855) -> (19.8755, 36.3855)
  arc A2891 (16.7005, 28.4798) -> (16.7005, 28.5433) centre (16.7005, 28.5115) ccw
  arc A2892 (16.4148, 27.6225) -> (16.4782, 27.6225) centre (16.4465, 27.6225) ccw
  arc A2893 (17.0498, 27.3685) -> (17.1133, 27.3685) centre (17.0816, 27.3685) ccw
  arc A2894 (16.4148, 28.2575) -> (16.4782, 28.2575) centre (16.4465, 28.2575) ccw
  line L891 (17.0815, 27.3685) -> (16.7005, 27.3685)
  arc A2895 (15.6845, 27.4002) -> (15.6845, 27.3368) centre (15.6845, 27.3685) ccw
  arc A2896 (15.8276, 27.8721) -> (15.7954, 27.8174) centre (15.8115, 27.8448) ccw
  arc A2897 (15.3353, 28.2575) -> (15.4623, 28.0353) centre (15.5932, 28.2575) ccw
  arc A2898 (15.367, 28.2575) -> (15.3035, 28.2575) centre (15.3353, 28.2575) ccw
  line L892 (15.8115, 27.8448) -> (15.4623, 28.0353)
  arc A2899 (15.7963, 27.8169) -> (15.8267, 27.8726) centre (15.8115, 27.8448) ccw
  arc A2900 (17.1133, 28.0035) -> (17.0498, 28.0035) centre (17.0816, 28.0035) ccw
  arc A2901 (15.9385, 27.6225) -> (15.8115, 27.8448) centre (15.6805, 27.6225) ccw
  arc A2902 (16.7005, 28.5433) -> (16.7005, 28.4798) centre (16.7005, 28.5115) ccw
  line L893 (17.6276, 28.2575) -> (17.9451, 28.5115)
  arc A2903 (15.6845, 27.3685) -> (15.9385, 27.6225) centre (15.6845, 27.6225) ccw
  arc A2904 (17.6276, 27.4002) -> (17.6276, 27.3368) centre (17.6276, 27.3685) ccw
  arc A2905 (20.5931, 35.2425) -> (20.6565, 35.2425) centre (20.6248, 35.2425) ccw
  line L894 (20.3073, 35.2425) -> (20.9423, 35.2425)
  arc A2906 (17.9768, 28.5115) -> (17.9134, 28.5115) centre (17.9451, 28.5115) ccw
  arc A2907 (19.2405, 36.4173) -> (19.2405, 36.3537) centre (19.2405, 36.3855) ccw
  arc A2908 (19.5897, 36.3855) -> (19.5263, 36.3855) centre (19.558, 36.3855) ccw
  arc A2909 (20.3073, 35.2743) -> (20.3073, 35.2107) centre (20.3073, 35.2425) ccw
  arc A2910 (20.9423, 35.2107) -> (20.9423, 35.2743) centre (20.9423, 35.2425) ccw
  arc A2911 (19.8755, 36.3537) -> (19.8755, 36.4173) centre (19.8755, 36.3855) ccw